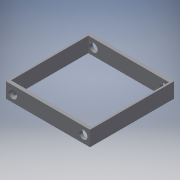
# Autodesk Inventor part: Hoofdplaat zijkant
Saved by Autodesk Inventor 2018.3 (Build 223284000, 284)
## iProperties
Created: 2020-11-23
Part Number: Hoofdplaat zijkant
Material: Generic
Document SubType Name: Modeling
Designer: daanv
Density: 1 g/cm^3
Appearance: Default
Author: daanv
Autodesk Inventor part; units mm, degrees
ref_plane "YZ Plane" through (0, 0, 0) normal (1, 0, 0) x (0, 1, 0)
ref_plane "XZ Plane" through (0, 0, 0) normal (0, 1, 0) x (-1, 0, 0)
ref_plane "XY Plane" through (0, 0, 0) normal (0, 0, 1) x (1, 0, 0)
sketch "Sketch1" plane through (0, 0, 0) normal (0, 0, 1) x (1, 0, 0)
  line L0 (0, 0) -> (0, 50)
  line L1 (0, 50) -> (50, 50)
  line L2 (50, 50) -> (50, 0)
  line L3 (50, 0) -> (0, 0)
  line L4 (1, 1) -> (1, 49)
  line L5 (1, 49) -> (49, 49)
  line L6 (49, 49) -> (49, 1)
  line L7 (49, 1) -> (1, 1)
  dimension "d0" = 50
  dimension "d1" = 50
  dimension "d2" = 48
  dimension "d3" = 48
  constraints: 16 end point, 6 perpendicular, 2 vertical
  measures "d0" distance of L0.start L0.end
  measures "d1" distance of L0.end L1.end
  measures "d2" distance of L4.start L4.end
  measures "d3" distance of L4.end L5.end
extrude "Extrusion1" add sketch "Sketch1" along normal blind 9
sketch "Sketch2" plane through (1, 49, 0) normal (0, -1, 0) x (1, 0, 0)
  line L0 (48, 0) -> (0, 0) projected
  line L1 (48, 0) -> (48, 9) projected
  line L2 (0, 9) -> (48, 9) projected
  line L3 (0, 0) -> (0, 9) projected
  point P0 (-1, 0)
extrude "Extrusion2" add sketch "Sketch2" along normal blind 1
sketch "Sketch3" plane through (1, 1, 0) normal (0, 1, 0) x (1, 0, 0)
  line L0 (0, 0) -> (48, 0) projected
  line L1 (0, 0) -> (0, -9) projected
  line L2 (48, -9) -> (0, -9) projected
  line L3 (48, 0) -> (48, -9) projected
  point P0 (-1, 0)
extrude "Extrusion3" add sketch "Sketch3" along normal blind 1
sketch "Sketch4" plane through (0, 50, 0) normal (0, 1, 0) x (1, 0, 0)
  point P0 (4, -4.3741)
  point P1 (46, -4.5)
hole "Hole1" at (4, 50, 4.3741) at (46, 50, 4.5) direction (0, -1, 0) diameter 5 end through all
body "Solid1"
